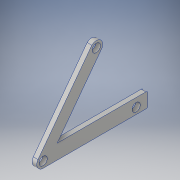
# Autodesk Inventor part: Marco_trasero_triciclo
Saved by Autodesk Inventor 2019 (Build 230136000, 136)
## iProperties
Created: 2019-11-14
Part Number: Marco_trasero_triciclo
Material: Aluminum 6061
Document SubType Name: Modeling
Designer: Domenico
Density: 2.7 g/cm^3
Appearance: Aluminum - Flat
Author: Domenico
Autodesk Inventor part; units mm, degrees
ref_plane "YZ Plane" through (0, 0, 0) normal (1, 0, 0) x (0, 1, 0)
ref_plane "XZ Plane" through (0, 0, 0) normal (0, 1, 0) x (-1, 0, 0)
ref_plane "XY Plane" through (0, 0, 0) normal (0, 0, 1) x (1, 0, 0)
sketch "Sketch1" plane through (0, 0, 0) normal (1, 0, 0) x (0, 1, 0)
  line L0 (0, 0) -> (0, 201.966)
  circle A0 centre (12.3, 22.683) radius 7.95
  line L1 (0, 0) -> (16.4683, 0)
  circle A1 centre (12.3, 201.966) radius 7.95
  line L2 (0, 0) -> (28.5, 0)
  line L3 (28.5, 0) -> (28.5, 174.8193)
  line L4 (12.3, 22.683) -> (149.7256, 99.4246) construction
  circle A2 centre (149.7256, 99.4246) radius 7.95
  line L5 (28.5, 174.8193) -> (141.0282, 90.7272)
  arc A3 (141.0282, 90.7272) -> (158.423, 108.122) centre (149.7256, 99.4246) ccw
  line L6 (149.7256, 99.4246) -> (158.423, 108.122) construction
  line L7 (149.7256, 99.4246) -> (141.0282, 90.7272) construction
  line L8 (158.423, 108.122) -> (19.517, 211.9262)
  arc A4 (19.517, 211.9262) -> (0, 201.966) centre (12.3, 201.966) ccw
  dimension "d0" = 201.966
  dimension "d1" = 22.683
  dimension "d2" = 12.3
  dimension "d3" = 15.9
  dimension "d4" = 15.9
  dimension "d5" = 28.5
  dimension "d6" = 157.401
  dimension "d7" = 119.18
  dimension "d8" = 15.9
  dimension "d10" = 180
  dimension "d11" = 12.3
  dimension "d12" = 12.3
  dimension "d13" = 9.9602
  constraints: 18 end point, 5 centre point, 4 point on circle, 3 coincident, 2 horizontal, 1 horizontal alignment, 1 parallel, 1 perpendicular, 1 vertical, 1 vertical alignment
  measures "d0" distance of L0.start L0.end
  measures "d1" distance from line of L1 L4.start
  measures "d2" distance from line of L0 L4.start
  measures "d3" diameter of A0
  measures "d4" diameter of A1
  measures "d5" distance of L0.start L2.end
  measures "d6" distance of L4.start L4.end
  measures "d7" angle of L4 L3
  measures "d8" diameter of A2
  measures "d10" angle of L7 L6
  measures "d11" distance of L0.end A1.centre
  measures "d12" distance of L6.end L6.start
  measures "d13" vertical distance of A1.centre L8.end
extrude "Extrusion1" add sketch "Sketch1" along normal blind 9
fillet "Fillet1" radius 4 2 edges at (4.5, 28.5, 0) (4.5, 0, 0)
equation "\"d2\" = altura_hoyo"
equation "\"d3\" = D_eje"
equation "\"d4\" = D_eje"
equation "\"d6\" = d_entre_ejes"
equation "\"d8\" = D_eje"
equation "\"d12\" = d11"
equation "\"altura_hoyo\" = 12.3"
equation "\"D_eje\" = 15.9"
equation "\"d_entre_ejes\" = 157.401"
body "Solid1"
